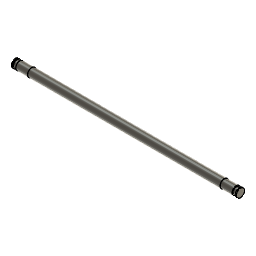
Battle bot 150 mm v15 (Autodesk Fusion 360 archive; units mm, degrees)
design "wedge pin"
Autodesk Fusion 360 part; units mm, degrees
sketch "Sketch1" plane through (0, 0, 0) normal (1, 0, 0) x (0, 1, 0)
  circle A0 centre (0, 0) radius 3.9
  dimension "d1" = 7.8
  constraint coincident A0.centre origin
  measures "d1" diameter of A0
extrude "Extrude1" add sketch "Sketch1" along normal mid plane 200
sketch "Sketch2" plane through (0, 0, 0) normal (0, 1, 0) x (1, 0, 0)
  line L0 (100, -3.9) -> (100, -2.9)
  line L1 (100, -2.9) -> (103, -2.9)
  line L2 (103, -2.9) -> (103, -3.9)
  line L3 (103, -3.9) -> (104, -3.9)
  line L4 (104, -3.9) -> (104, 0)
  line L5 (104, 0) -> (100, 0)
  line L6 (100, 0) -> (100, -2.9)
  dimension "d7" = 3
  constraint vertical L0
  constraint perpendicular L0 L1
  constraint perpendicular L1 L2
  constraint perpendicular L2 L3
  constraint perpendicular L3 L4
  constraint perpendicular L4 L5
  constraint perpendicular L1 L6
  measures "d7" distance of L0.end L1.end
revolve "Revolve1" add sketch "Sketch2" angle 360 about axis through (104, 0, 0) along (-1, 0, 0)
mirror "Mirror1" about plane through (0, 0, 0) normal (1, 0, 0) of "Revolve1"
sketch "Sketch3" plane through (-104, 0, 0) normal (-1, 0, 0) x (0, -1, 0)
  circle A0 centre (0, 0) radius 3.8
  circle A1 centre (0, 0) radius 3.9
  constraint coincident A0.centre A1.centre
  constraint concentric A0 A1
extrude "Extrude2" cut sketch "Sketch3" against normal blind 15
mirror "Mirror2" about plane through (0, 0, 0) normal (1, 0, 0) of "Extrude2"
named bodies: "wedge pin"

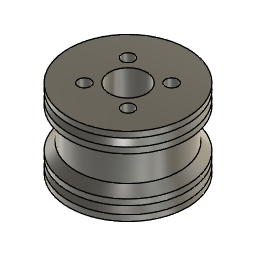
design "DMI battlebot lego rubber adapter"
Autodesk Fusion 360 part; units mm, degrees
sketch "Sketch1" plane through (0, 0, 0) normal (1, 0, 0) x (0, 1, 0)
  line L0 (15.2, 10) -> (-15.2, 10)
  line L1 (-15.2, 10) -> (-15.2, -10)
  line L2 (-15.2, -10) -> (15.2, -10)
  line L3 (15.2, -10) -> (15.2, 10)
  line L4 (15.2, 10) -> (-15.2, -10) construction
  line L5 (-15.2, 10) -> (15.2, -10) construction
  line L6 (0, 10) -> (0, -10)
  line L7 (15.2, 10) -> (15.2, 8.5)
  line L8 (15.2, 8.5) -> (13.7, 8.5)
  line L9 (13.7, 8.5) -> (13.7, 6.5)
  line L10 (13.7, 6.5) -> (15.2, 6.5)
  line L11 (15.2, -10) -> (15.2, -8.5)
  line L12 (15.2, -8.5) -> (13.7, -8.5)
  line L13 (13.7, -8.5) -> (13.7, -6.5)
  line L14 (13.7, -6.5) -> (15.2, -6.5)
  line L15 (15.2, -6.5) -> (15.2, -5)
  line L16 (15.2, -5) -> (13.2, -5)
  line L17 (15.2, 6.5) -> (15.2, 5)
  line L18 (15.2, 5) -> (13.2, 5)
  line L19 (13.2, 5) -> (13.2, -5)
  dimension "d1" = 30.4
  dimension "d2" = 20
  dimension "d3" = 1.5
  dimension "d4" = 1.5
  dimension "d5" = 2
  dimension "d6" = 1.5
  dimension "d7" = 1.5
  dimension "d8" = 2
  dimension "d9" = 1.5
  dimension "d10" = 2
  dimension "d11" = 2
  constraint horizontal L0
  constraint perpendicular L0 L1
  constraint parallel L0 L2
  constraint parallel L1 L3
  constraint coincident L4 origin
  constraint coincident L5 origin
  constraint midpoint L0 L6.start
  constraint midpoint L2 L6.end
  constraint perpendicular L0 L7
  constraint perpendicular L7 L8
  constraint perpendicular L8 L9
  constraint coincident L3 L10.end
  constraint perpendicular L3 L10
  constraint perpendicular L2 L11
  constraint perpendicular L3 L12
  constraint perpendicular L12 L13
  constraint coincident L3 L14.end
  constraint perpendicular L3 L14
  constraint perpendicular L14 L15
  constraint perpendicular L3 L16
  constraint coincident L3 L17.end
  constraint perpendicular L3 L18
  constraint perpendicular L16 L19
  measures "d1" distance of L1.end L2.end
  measures "d2" distance of L0.end L1.end
  measures "d3" distance of L0.start L7.end
  measures "d4" distance of L7.end L8.end
  measures "d5" distance of L8.end L9.end
  measures "d6" distance of L2.end L11.end
  measures "d7" distance of L11.end L12.end
  measures "d8" distance of L12.end L13.end
  measures "d9" distance of L14.end L15.end
  measures "d10" distance of L15.end L16.end
  measures "d11" distance of L17.end L18.end
revolve "Revolve1" add sketch "Sketch1" angle 360 about axis through (0, 0, 10) along (0, 0, -1) contours L0 L2 L3 L6 L7 L8 L9 L10 L11 L12 L13 L14 L15 L16 L17 L18 L19
sketch "Sketch2" plane through (0, 0, 10) normal (0, 0, 1) x (-1, 0, 0)
  circle A0 centre (0, 0) radius 15.2
  line L0 (5.588, -5.588) -> (-5.588, -5.588)
  line L1 (-5.588, -5.588) -> (-5.588, 5.588)
  line L2 (-5.588, 5.588) -> (5.588, 5.588)
  line L3 (5.588, 5.588) -> (5.588, -5.588)
  line L4 (5.588, -5.588) -> (-5.588, 5.588) construction
  line L5 (-5.588, -5.588) -> (5.588, 5.588) construction
  circle A1 centre (5.588, -5.588) radius 1.5875
  dimension "d13" = 11.176
  dimension "d14" = 11.176
  dimension "d15" = 3.175
  constraint horizontal L0
  constraint perpendicular L0 L1
  constraint parallel L0 L2
  constraint parallel L1 L3
  constraint coincident L4 A0.centre
  constraint coincident L5 A0.centre
  constraint coincident A0.centre origin
  constraint coincident L0.start L3.end
  measures "d13" distance of L1.end L2.end
  measures "d14" distance of L0.end L1.end
  measures "d15" diameter of A1
extrude "Extrude1" cut sketch "Sketch2" against normal blind 25 contours L0 L3 A1 | L0 L3 A1
pattern_circular "C-Pattern1" count 4 over 360 about axis through (0, 0, 1.75) along (0, 0, 1) of "Extrude1"
chamfer "Chamfer1" distance 1.5 angle 45 1 edges at (-12.7729, 4.9541, -8.5)
chamfer "Chamfer2" distance 2 angle 45 1 edges at (-12.3067, 4.7733, -5)
chamfer "Chamfer3" distance 1.5 angle 45 1 edges at (-12.7729, 4.9541, 6.5)
sketch "Sketch3" plane through (0, 0, -10) normal (0, 0, -1) x (1, 0, 0)
  circle A0 centre (5.588, -5.588) radius 1.5875
  circle A1 centre (5.588, 5.588) radius 1.5875
  circle A2 centre (-5.588, 5.588) radius 1.5875
  circle A3 centre (-5.588, -5.588) radius 1.5875
  circle A4 centre (0, 0) radius 15.2
  circle A5 centre (-5.588, 5.588) radius 2.5
  circle A6 centre (-5.588, -5.588) radius 2.5
  circle A7 centre (5.588, -5.588) radius 2.5
  circle A8 centre (5.588, 5.588) radius 2.5
  dimension "d23" = 5
  dimension "d24" = 5
  dimension "d25" = 5
  dimension "d26" = 5
  constraint concentric A2 A5
  constraint concentric A3 A6
  constraint concentric A0 A7
  constraint concentric A1 A8
  measures "d23" diameter of A5
  measures "d24" diameter of A6
  measures "d25" diameter of A7
  measures "d26" diameter of A8
extrude "Extrude2" cut sketch "Sketch3" against normal blind 15 contours A5 | A6 | A7 | A8
sketch "Sketch4" plane through (0, 0, 10) normal (0, 0, 1) x (-1, 0, 0)
  circle A0 centre (-5.588, -5.588) radius 1.5875
  circle A1 centre (-5.588, 5.588) radius 1.5875
  circle A2 centre (5.588, 5.588) radius 1.5875
  circle A3 centre (5.588, -5.588) radius 1.5875
  circle A4 centre (0, 0) radius 15.2
  circle A5 centre (0, 0) radius 4.7625
  dimension "d29" = 9.525
  constraint coincident A4.centre A5.centre
  measures "d29" diameter of A5
extrude "Extrude3" cut sketch "Sketch4" against normal blind 26 contours A5
equation "d13 = 0.315 in + 0.125 in"
equation "d14 = 0.315 in + 0.125 in"
named bodies: "wheel adapter"
